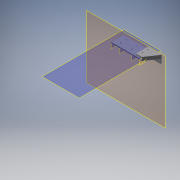
# Autodesk Inventor part: SidePlateMount
Saved by Autodesk Inventor 2016 (Build 200138000, 138)
## iProperties
Created: 2016-04-23
Part Number: SidePlateMount
Material: Generic
Document SubType Name: Modeling
Designer: Scott
Density: 1 g/cm^3
Appearance: Default
Author: Scott
Autodesk Inventor part; units mm, degrees
ref_plane "YZ Plane" through (0, 0, 0) normal (1, 0, 0) x (0, 1, 0)
ref_plane "XZ Plane" through (0, 0, 0) normal (0, 1, 0) x (-1, 0, 0)
ref_plane "Work Plane1" through (0, 0, 0) normal (0, 0, 1) x (1, 0, 0)
sketch "Sketch1" plane through (0, 0, 0) normal (0, 0, 1) x (1, 0, 0)
  circle A0 centre (15.875, 121.204) radius 2.2225 projected
  circle A1 centre (66.675, 121.204) radius 2.2225 projected
  circle A2 centre (117.475, 121.204) radius 2.2225 projected
  line L0 (168.275, -133.904) -> (168.275, 133.904) projected
  line L1 (-34.925, 108.504) -> (168.275, 108.504)
  line L2 (168.275, 108.504) -> (168.275, 133.904)
  line L3 (168.275, 133.904) -> (-34.925, 133.904)
  line L4 (-34.925, 133.904) -> (-34.925, 108.504)
  line L5 (-34.925, 108.504) -> (168.275, 133.904) construction
  line L6 (168.275, 108.504) -> (-34.925, 133.904) construction
  point P0 (0, 0)
  constraints: 12 end point, 2 midpoint, 2 parallel, 1 horizontal, 1 perpendicular
extrude "Extrusion1" add sketch "Sketch1" along normal blind 5.08
ref_plane "Work Plane2" through (69.756404, 133.918249, 155.730615) normal (0.0006325, -0.9999998, 0) x (0.9999998, 0.0006325, 0.0000106)
sketch "Sketch2" plane through (69.756404, 133.918249, 155.730615) normal (0.0006325, -0.9999998, 0) x (0.9999998, 0.0006325, 0.0000106)
  ellipse E0 centre (44.439887, 35.022911) end of major axis (44.439864, 32.800411) minor radius 2.2225
  ellipse E1 centre (44.439482, -3.077089) end of major axis (44.439459, -5.299589) minor radius 2.2225
  ellipse E2 centre (-3.815566, -117.630576) end of major axis (-3.815542, -115.408076) minor radius 2.2225
  ellipse E3 centre (46.984159, -143.031116) end of major axis (46.984182, -140.808616) minor radius 2.2225
  ellipse E4 centre (-54.61583, -143.030036) end of major axis (-54.615807, -140.807536) minor radius 2.2225
  ellipse E5 centre (-3.815836, -143.030576) end of major axis (-3.815812, -140.808076) minor radius 2.2225
  ellipse E6 centre (46.984429, -117.631116) end of major axis (46.984452, -115.408616) minor radius 2.2225
  ellipse E7 centre (-54.61556, -117.630036) end of major axis (-54.615537, -115.407536) minor radius 2.2225
  ellipse E8 centre (15.283791, 124.972429) end of major axis (15.283738, 119.972429) minor radius 4.999999
  ellipse E9 centre (15.284236, 166.850251) end of major axis (15.284194, 162.850251) minor radius 4
  ellipse E10 centre (15.283346, 83.094607) end of major axis (15.283303, 79.094607) minor radius 4
  ellipse E11 centre (-10.115761, 166.850521) end of major axis (-10.115788, 164.310521) minor radius 2.54
  ellipse E12 centre (-10.109874, 83.253753) end of major axis (-10.109901, 80.713753) minor radius 2.54
  ellipse E13 centre (40.682106, 166.521487) end of major axis (40.682079, 163.981487) minor radius 2.54
  ellipse E14 centre (41.130544, 83.243775) end of major axis (41.130517, 80.703775) minor radius 2.54
  line L0 (63.491506, 187.422709) -> (-25.408484, 187.423654)
  line L1 (-25.408484, 187.423654) -> (-95.26219, -161.825603)
  line L2 (-95.26219, -161.825603) -> (63.487792, -161.827291)
  line L3 (63.487792, -161.827291) -> (63.491506, 187.422709)
  line L4 (-54.61556, -117.630036) -> (-54.61556, -98.580036)
  line L5 (-54.61556, -98.580036) -> (-82.612379, -98.580036)
  line L6 (-82.612379, -98.580036) -> (63.488465, -98.580036)
  point P0 (-69.842744, -155.729873)
  dimension "d2" = 19.05
  constraints: 6 end point, 3 point on line, 1 perpendicular, 1 vertical, 15 other
  measures "d2" distance of L4.start L4.end
extrude "Extrusion2" add sketch "Sketch2" along normal blind 5.08 contours L3 L2 L1 L5 L6
sketch "Sketch3" plane through (0, 0, 5.08) normal (0, 0, 1) x (1, 0, 0)
  circle A0 centre (155.575, 121.204) radius 2.2225 projected
  point P0 (0, 0)
extrude "Extrusion3" cut sketch "Sketch3" along normal mid plane 25.4
sketch "Sketch4" plane through (69.759617, 128.83825, 155.730615) normal (0.0006325, -0.9999998, 0) x (0.9999998, 0.0006325, 0.0000106)
  line L0 (63.488465, -98.580036) -> (-82.612379, -98.580036)
  line L1 (98.516965, -150.651662) -> (63.487911, -150.65129)
  line L2 (-104.699058, -150.649501) -> (98.500901, -150.651662)
  line L3 (98.500901, -150.651662) -> (63.488465, -98.580036)
  line L4 (98.500901, -150.651662) -> (98.516965, -150.651662)
  line L5 (98.516965, -150.651662) -> (98.516965, -155.729873)
  line L6 (63.487911, -150.65129) -> (63.488465, -98.580036)
  line L7 (63.488465, -98.580036) -> (63.487911, -150.65129)
  line L8 (63.487911, -150.65129) -> (98.500901, -150.651662)
  line L9 (63.487857, -155.73129) -> (63.487911, -150.65129)
  line L10 (98.516965, -150.651662) -> (63.487911, -150.65129)
  line L11 (98.516911, -155.731662) -> (98.516965, -150.651662)
  line L12 (63.487857, -155.73129) -> (98.516911, -155.731662)
  point P0 (-69.842744, -155.729873)
  constraints: 8 end point, 1 collinear, 1 perpendicular, 1 vertical
ref_plane "Work Plane3" through (-25.357797, 139.954093, -6.097175) normal (-0.0006325, 0.9999998, 0) x (-0.0000106, 0, 1)
extrude "Extrusion4" add sketch "Sketch4" against normal up to surface (11.176 mm away)
sketch "Sketch5" plane through (133.242049, 140.054401, 57.151254) normal (-0.0006325, 0.9999998, 0) x (0.9999998, 0.0006325, 0)
  line L0 (0, 57.151254) -> (35.029054, 57.151254)
  line L1 (0, 0) -> (0, 57.151254)
  line L2 (35.01299, 52.071254) -> (0, 0)
  line L3 (35.029054, 52.071254) -> (35.01299, 52.071254)
  line L4 (35.029054, 57.151254) -> (35.029054, 52.071254)
  line L5 (35.01299, 57.151254) -> (35.01299, 52.071254)
  line L6 (35.01299, 57.151254) -> (-28.48701, 57.151254)
  line L7 (-157.530782, 57.151254) -> (0, 57.151254)
  line L8 (-28.48701, 57.151254) -> (-28.48701, 0.000303)
  line L9 (0, 0) -> (-146.100843, 0.001553)
  line L10 (0, 0) -> (-28.48701, 0.000303)
  circle A0 centre (-16.352604, 19.051254) radius 2.2225
  circle A1 centre (-16.352604, 44.451254) radius 2.2225
  point P0 (-133.330601, 57.151255)
  dimension "d9" = 63.5
  constraints: 6 end point, 2 point on line, 1 collinear, 1 perpendicular
  measures "d9" distance of L5.start L6.end
extrude "Extrusion5" add sketch "Sketch5" along normal blind 5.08 contours L0 L5 L2 L1 | L1 L9 L8 L6
ref_plane "Work Plane4" through (133.249117, 128.878404, 57.151254) normal (1, 0, 0) x (0, 1, 0)
sketch "Sketch6" plane through (133.249117, 128.878404, 57.151254) normal (1, 0, 0) x (0, 1, 0)
  line L0 (-0.092403, -0.001553) -> (-0.098989, -52.071254)
  line L1 (5.025597, -52.071254) -> (-20.374403, -52.071254)
  line L2 (-0.092403, -0.001553) -> (-20.374403, -52.071254)
  point P0 (-128.878404, -57.151254)
  constraints: 2 end point
extrude "Extrusion6" add sketch "Sketch6" against normal blind 5.08
ref_plane "Work Plane6" through (29.744117, 128.878404, 57.151254) normal (-1, 0, 0) x (0, 0, 1)
ref_plane "Work Plane5" through (86.894117, 128.878404, 57.151254) normal (-1, 0, 0) x (0, 0, 1)
sketch "Sketch7" plane through (86.894117, 128.878404, 57.151254) normal (-1, 0, 0) x (0, 0, 1)
  line L0 (-0.001553, -0.092403) -> (-52.071254, -0.098989)
  line L1 (-52.071254, -20.374403) -> (-52.071254, -0.098989)
  line L2 (-52.071254, -20.374403) -> (-0.001553, -0.092403)
  point P0 (-57.151254, -128.878404)
extrude "Extrusion7" add sketch "Sketch7" along normal mid plane 5.08
sketch "Sketch8" plane through (29.744117, 128.878404, 57.151254) normal (-1, 0, 0) x (0, 0, 1)
  line L0 (-0.001553, -0.092403) -> (-52.071254, -0.098989)
  line L1 (-52.071254, -20.374403) -> (-52.071254, -0.098989)
  line L2 (-52.071254, -20.374403) -> (-0.001553, -0.092403)
  point P0 (-57.151254, -128.878404)
extrude "Extrusion8" add sketch "Sketch8" against normal blind 5.08
ref_plane "Work Plane7" through (-9.943383, 128.878404, 57.151254) normal (-1, 0, 0) x (0, 0, 1)
sketch "Sketch9" plane through (-9.943383, 128.878404, 57.151254) normal (-1, 0, 0) x (0, 0, 1)
  line L0 (-0.001553, -0.092403) -> (-52.071254, -0.098989)
  line L1 (-52.071254, -20.374403) -> (-52.071254, -0.098989)
  line L2 (-52.071254, -20.374403) -> (-0.001553, -0.092403)
  point P0 (-57.151254, -128.878404)
extrude "Extrusion9" add sketch "Sketch9" against normal blind 5.08
chamfer "Chamfer1" distance 22.225 angle 45 1 edges at (-34.925, 108.504, 2.54)
sketch "Sketch10" plane through (69.759617, 128.83825, 155.730615) normal (0.0006325, -0.9999998, 0) x (0.9999998, 0.0006325, 0.0000106)
  line L0 (-94.042925, -155.729615) -> (63.487857, -155.73129)
  line L1 (-95.26219, -161.825603) -> (63.487792, -161.827291)
  line L2 (-94.042925, -155.729615) -> (-95.26219, -161.825603)
  line L3 (63.487792, -161.827291) -> (63.487857, -155.73129)
  line L4 (-104.685002, -150.649501) -> (-104.685056, -155.729501)
  line L5 (-104.683048, -155.729501) -> (-104.682994, -150.649501)
  line L6 (-82.474063, -150.649738) -> (-104.685002, -150.649501)
  line L7 (-104.685056, -155.729501) -> (-82.474117, -155.729738)
  line L8 (-74.624066, -98.580121) -> (-74.637447, -150.649821)
  line L9 (-79.704065, -98.580067) -> (-79.704623, -150.649767)
  line L10 (-82.612379, -98.580036) -> (-93.026871, -150.649625)
  line L11 (-79.704623, -150.649767) -> (-79.704677, -155.729767)
  line L12 (-79.704623, -150.649767) -> (-79.704677, -155.729767)
  line L13 (-93.026871, -150.649625) -> (-22.528764, -150.650375)
  line L14 (-82.612379, -98.580036) -> (-79.704065, -98.580067)
  point P0 (-69.842744, -155.729873)
  constraints: 6 end point, 2 perpendicular, 1 point on line
extrude "Extrusion10" cut sketch "Sketch10" along normal mid plane 254 contours L7 L5 L6 L13 L11 L0 | L0 L3 L1 L2 | L13 L6 L10 L14 L9
body "Solid1"
